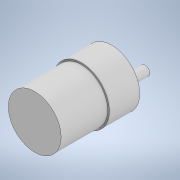
# Autodesk Inventor part: ShootingMech_Moter
Saved by Autodesk Inventor 2020 (Build 240168000, 168)
## iProperties
Created: 2022-01-27
Part Number: ShootingMech_Moter
Material: Generic
Document SubType Name: Modeling
Designer: danie
Density: 1 g/cm^3
Appearance: Default
Author: danie
Autodesk Inventor part; units mm, degrees
ref_plane "YZ Plane" through (0, 0, 0) normal (1, 0, 0) x (0, 1, 0)
ref_plane "XZ Plane" through (0, 0, 0) normal (0, 1, 0) x (-1, 0, 0)
ref_plane "XY Plane" through (0, 0, 0) normal (0, 0, 1) x (1, 0, 0)
sketch "Sketch1" plane through (0, 0, 0) normal (0, 0, 1) x (1, 0, 0)
  circle A0 centre (0, 0) radius 17.399
  dimension "d0" = 34.798
  constraints: 1 centre point, 1 coincident
  measures "d0" diameter of A0
extrude "Extrusion1" add sketch "Sketch1" against normal blind 30.734
sketch "Sketch2" plane through (0, 0, -30.734) normal (0, 0, -1) x (-1, 0, 0)
  circle A0 centre (0, 0) radius 18.415
  dimension "d3" = 36.83
  constraints: 1 centre point, 1 coincident
  measures "d3" diameter of A0
extrude "Extrusion2" add sketch "Sketch2" along normal blind 20.066
sketch "Sketch3" plane through (0, 0, -50.8) normal (0, 0, -1) x (-1, 0, 0)
  line L0 (0, 0) -> (0, -7.112) construction
  circle A0 centre (0, -7.112) radius 5.969
  dimension "d6" = 7.112
  dimension "d7" = 11.938
  constraints: 2 end point, 1 centre point, 1 coincident, 1 vertical
  measures "d6" distance of L0.start L0.end
  measures "d7" diameter of A0
extrude "Extrusion3" add sketch "Sketch3" along normal blind 6.096
sketch "Sketch4" plane through (0, -7.112, -56.896) normal (0, 0, -1) x (-1, 0, 0)
  circle A0 centre (0, 0) radius 3.048
  point P0 (0, 7.112)
  dimension "d10" = 6.096
  constraints: 1 centre point
  measures "d10" diameter of A0
extrude "Extrusion4" add sketch "Sketch4" along normal blind 16.002
body "Solid1"
